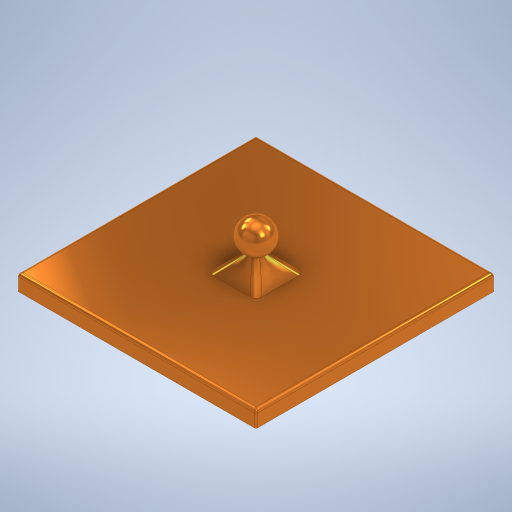
# Autodesk Inventor part: coffee container lock
Saved by Autodesk Inventor 2023 (Build 270158000, 158)
## iProperties
Created: 2022-11-26
Part Number: coffee container lock
Material: Gold
Document SubType Name: Modeling
Designer: abdul
Density: 19.3 g/cm^3
Appearance: Metal 1600F Hot
Author: abdul
Autodesk Inventor part; units mm, degrees
ref_plane "YZ Plane" through (0, 0, 0) normal (1, 0, 0) x (0, 1, 0)
ref_plane "XZ Plane" through (0, 0, 0) normal (0, 1, 0) x (-1, 0, 0)
sketch "Sketch1" plane through (0, 0, 0) normal (0, 1, 0) x (-1, 0, 0)
  line L0 (75, 75) -> (-75, 75)
  line L1 (-75, 75) -> (-75, -75)
  line L2 (-75, -75) -> (75, -75)
  line L3 (75, -75) -> (75, 75)
  point P0 (0, 0)
  dimension "d0" = 150
  dimension "d1" = 150
  dimension "d2" = 75
  dimension "d3" = 75
  constraints: 8 end point, 2 parallel, 1 horizontal, 1 perpendicular
  measures "d0" distance of L2.end L1.end
  measures "d1" distance of L1.end L0.end
  measures "d2" distance from line of L0 point (0, 0)
  measures "d3" distance from line of point (0, 0) L3
extrude "Extrusion1" add sketch "Sketch1" along normal blind 10
ref_plane "Work Plane1" through (0, 30, 0) normal (0, 1, 0) x (1, 0, 0)
sketch "Sketch5" plane through (0, 30, 0) normal (0, 1, 0) x (1, 0, 0)
  line L0 (-10, 0) -> (10, 0)
  arc A0 (-10, 0) -> (10, 0) centre (0, 0) ccw
  point P0 (0, 0)
  point P1 (0, 0)
  dimension "d7" = 20
  dimension "d8" = 10
  constraints: 2 end point, 2 point on circle, 1 centre point, 1 coincident, 1 horizontal, 1 midpoint
  measures "d7" distance of L0.start L0.end
  measures "d8" radius of A0
revolve "Revolution1" add sketch "Sketch5" angle 360 about axis through (-10, 30, 0) along (1, 0, 0)
sketch "Sketch6" plane through (0, 10, 0) normal (0, 1, 0) x (1, 0, 0)
  line L0 (15, -15) -> (-15, -15)
  line L1 (-15, -15) -> (-15, 15)
  line L2 (-15, 15) -> (15, 15)
  line L3 (15, 15) -> (15, -15)
  point P0 (0, 0)
  point P1 (0, -15)
  point P2 (-15, 0)
  dimension "d10" = 30
  dimension "d11" = 30
  constraints: 8 end point, 2 midpoint, 2 parallel, 1 horizontal, 1 horizontal alignment, 1 perpendicular, 1 vertical alignment
  measures "d10" distance of L1.end L2.end
  measures "d11" distance of L0.end L1.end
ref_plane "Work Plane2" through (0, 22, 0) normal (0, 1, 0) x (1, 0, 0)
sketch "Sketch7" plane through (0, 22, 0) normal (0, 1, 0) x (1, 0, 0)
  circle A0 centre (0, 0) radius 4
  dimension "d14" = 8
  constraints: 1 centre point, 1 coincident
  measures "d14" diameter of A0
loft "Loft1" add profiles "Sketch6", "Sketch7"
fillet "Fillet1" radius 5 5 edges at (9.2575, 15.6615, 9.2575) (9.8694, 15.597, 0) (9.2575, 15.6615, -9.2575) (-9.2575, 15.6615, -9.2575) (-9.2575, 15.6615, 9.2575)
sketch "Sketch8" plane through (0, 0, 0) normal (0, -1, 0) x (1, 0, 0)
  line L0 (72.4, -72.4) -> (-72.4, -72.4)
  line L1 (-72.4, -72.4) -> (-72.4, 72.4)
  line L2 (-72.4, 72.4) -> (72.4, 72.4)
  line L3 (72.4, 72.4) -> (72.4, -72.4)
  line L4 (75, -75) -> (-75, -75) projected
  line L5 (75, 75) -> (75, -75) projected
  line L6 (-75, 75) -> (75, 75) projected
  line L7 (-75, -75) -> (-75, 75) projected
  point P0 (0, 0)
  dimension "d30" = 2.6
  dimension "d31" = 2.6
  dimension "d32" = 2.6
  dimension "d33" = 2.6
  constraints: 8 end point, 2 parallel, 1 horizontal, 1 perpendicular
  measures "d30" distance between parallel lines of L5 L3
  measures "d31" distance between parallel lines of L4 L0
  measures "d32" distance between parallel lines of L7 L1
  measures "d33" distance between parallel lines of L6 L2
extrude "Extrusion2" add sketch "Sketch8" along normal blind 2 contours L0 L1 L2 L3
fillet "Fillet2" radius 2 4 edges at (75, 10, 0) (0, 10, 75) (0, 10, -75) (-75, 10, 0)
fillet "Fillet3" radius 1 8 edges at (-74.4142, 9.4142, -74.4142) (-75, 4, -75) (74.4142, 9.4142, -74.4142) (75, 4, -75) (74.4142, 9.4142, 74.4142) (75, 4, 75) (-74.4142, 9.4142, 74.4142) (-75, 4, 75)
chamfer "Chamfer1" distance 0.5 angle 45 4 edges at (0, -2, -72.4) (-72.4, -2, 0) (0, -2, 72.4) (72.4, -2, 0)
body "Solid1"
